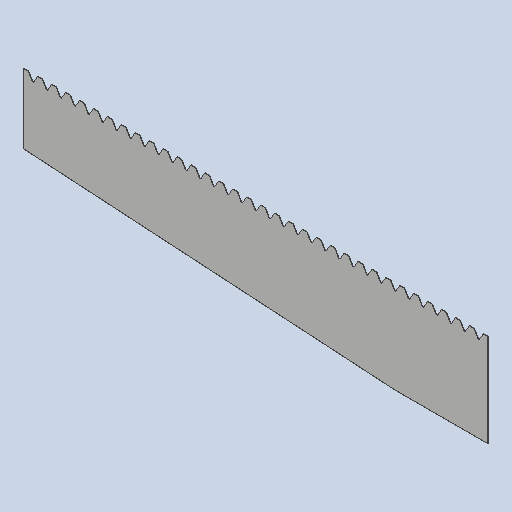
# Autodesk Inventor part: MSC 051 ridge 1
Saved by Autodesk Inventor 2024.2 (Build 282272000, 272)
## iProperties
Created: 2024-06-08
Part Number: MSC 051 ridge 1
Material: Generic
Document SubType Name: Sheet Metal
Designer: admin
Density: 1 g/cm^3
Appearance: Default
Sheet Metal Rule: Default
Stock Number: МОО 051 гребень 1
Author: admin
Autodesk Inventor part; units mm, degrees
ref_plane "YZ Plane" through (0, 0, 0) normal (1, 0, 0) x (0, 1, 0)
ref_plane "XZ Plane" through (0, 0, 0) normal (0, 1, 0) x (-1, 0, 0)
ref_plane "XY Plane" through (0, 0, 0) normal (0, 0, 1) x (1, 0, 0)
sketch "Sketch1" plane through (0, 0, 0) normal (0, 1, 0) x (-1, 0, 0)
  line L0 (0, 0) -> (0, -400)
  line L1 (2000, -300) -> (2000, 0)
  line L2 (2000, 0) -> (0, 0)
  line L3 (0, -400) -> (400, -400)
  line L4 (2000, -300) -> (400, -400)
  dimension "d0" = 400
  dimension "d1" = 2000
  dimension "d2" = 300
  dimension "d4" = 400
  measures "d0" distance of L0.start L0.end
  measures "d1" distance of L1.end L0.start
  measures "d2" distance of L1.start L1.end
  measures "d4" distance of L0.end L3.end
extrude "Plate1" add sketch "Sketch1" along normal blind 2
sketch "Sketch3" plane through (0, 0, 0) normal (0, -1, 0) x (1, 0, 0)
  line L0 (-2000, 0) -> (0, 0) projected
  line L1 (-20, 0) -> (-37.5, -30)
  line L2 (-37.5, -30) -> (-42.5, -30)
  line L3 (-42.5, -30) -> (-60, 0)
  dimension "d12" = 5
  dimension "d13" = 40
  dimension "d14" = 30
  dimension "d15" = 20
  constraints: 6 end point, 2 point on line, 1 equal length, 1 horizontal
  measures "d12" distance of L1.end L2.end
  measures "d13" distance of L1.start L3.end
  measures "d14" distance between parallel lines of L2 L0
  measures "d15" distance of L0.end L1.start
extrude "Extrusion2" cut sketch "Sketch3" against normal through all
fillet "Fillet2" radius 2 4 edges at (-20, 1, 0) (-37.5, 1, -30) (-42.5, 1, -30) (-60, 1, 0)
pattern_linear "Rectangular Pattern1" count 33 spacing 60 along (-1, 0, 0) of "Extrusion2", "Fillet2"
equation "\"d3\" = Thickness"
equation "\"BendRadius\" = Thickness"
equation "\"BendReliefWidth\" = Thickness"
equation "\"BendReliefDepth\" = 0.5 * Thickness"
equation "\"CornerReliefSize\" = 4 * Thickness"
equation "\"MinimumRemnant\" = 2 * Thickness"
equation "\"TransitionRadius\" = BendRadius"
equation "\"JacobiRadiusSize\" = BendRadius"
equation "\"GapSize\" = Thickness"
equation "\"Thickness\" = 2"
body "Solid1"
